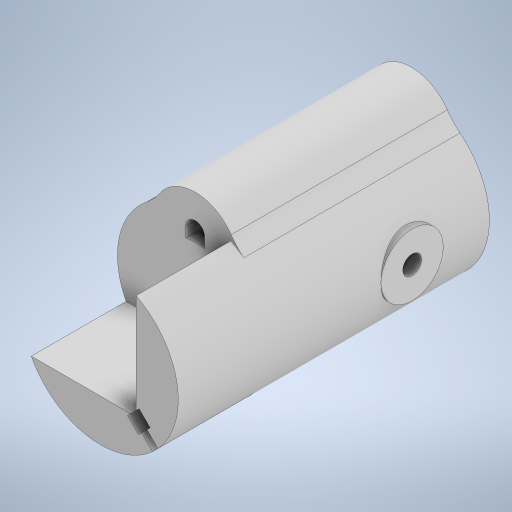
# Autodesk Inventor part: LandingFoot1
Saved by Autodesk Inventor 2023 (Build 270158000, 158)
## iProperties
Created: 2023-01-25
Part Number: LandingFoot1
Material: Generic
Document SubType Name: Modeling
Designer: chase
Density: 1 g/cm^3
Appearance: Default
Author: chase
Autodesk Inventor part; units mm, degrees
ref_plane "YZ Plane" through (0, 0, 0) normal (1, 0, 0) x (0, 1, 0)
ref_plane "XZ Plane" through (0, 0, 0) normal (0, 1, 0) x (-1, 0, 0)
ref_plane "XY Plane" through (0, 0, 0) normal (0, 0, 1) x (1, 0, 0)
sketch "Sketch1" plane through (0, 0, 0) normal (0, 0, 1) x (1, 0, 0)
  circle A0 centre (0, 0) radius 12.5
  dimension "d0" = 25
  constraints: 1 centre point
  measures "d0" diameter of A0
extrude "Extrusion1" add sketch "Sketch1" against normal blind 50
sketch "Sketch2" plane through (0, 0, 0) normal (0, 0, 1) x (1, 0, 0)
  circle A0 centre (0, 0) radius 12.5 projected
  line L0 (0, 12.5) -> (0, 0) construction
  line L1 (0, 0) -> (8.8388, -8.8388) construction
  line L2 (4.4548, -2.6163) -> (9.7581, -7.9196)
  line L3 (9.7581, -7.9196) -> (7.9196, -9.7581)
  line L4 (4.4548, -2.6163) -> (2.6163, -4.4548)
  line L5 (9.7581, -7.9196) -> (7.9196, -9.7581)
  line L6 (7.9903, -6.1518) -> (6.1518, -7.9903)
  line L7 (6.2225, -4.3841) -> (4.3841, -6.2225)
  line L8 (5.374, -4.5255) -> (4.5255, -5.374)
  line L9 (4.4194, -2.6517) -> (2.6517, -4.4194)
  line L10 (5.2679, -4.6315) -> (3.8537, -3.2173)
  line L11 (4.9497, -4.9497) -> (3.5355, -3.5355)
  line L12 (4.6315, -5.2679) -> (3.2173, -3.8537)
  line L13 (9.2631, -8.4146) -> (7.4953, -6.6468)
  line L14 (5.7276, -4.879) -> (5.374, -4.5255)
  line L15 (8.4146, -9.2631) -> (6.6468, -7.4953)
  line L16 (4.879, -5.7276) -> (4.5255, -5.374)
  line L17 (4.879, -5.7276) -> (-11.1106, -5.7276)
  line L18 (5.7276, -4.879) -> (5.7276, 11.1106)
  line L19 (3.8891, -5.7276) -> (2.6163, -4.4548)
  line L20 (7.9196, -9.7581) -> (7.8717, -9.7101)
  line L21 (6.1518, -7.9903) -> (4.3841, -6.2225)
  point P0 (7.955, -6.1872)
  point P1 (6.1872, -4.4194)
  point P2 (5.7276, -3.8891)
  point P3 (9.7101, -7.8717)
  point P4 (8.8388, -8.8388)
  dimension "d12" = 135
  dimension "d14" = 7.5
  dimension "d16" = 7.5
  dimension "d18" = 2.5
  dimension "d19" = 2.5
  dimension "d20" = 0.5
  dimension "d27" = 1.2
  dimension "d57" = 0.9
  dimension "d58" = 0.45
  dimension "d59" = 1.3
  constraints: 44 end point, 9 point on line, 6 parallel, 5 point on circle, 4 perpendicular, 2 collinear, 1 horizontal, 1 tangent, 1 vertical
  measures "d12" angle of L1 L0
  measures "d14" distance of L2.start L2.end
  measures "d16" distance of L3.end L4.end
  measures "d18" distance between parallel lines of L3 L6
  measures "d19" distance between parallel lines of L6 L7
  measures "d20" distance between parallel lines of L7 L8
  measures "d27" distance between parallel lines of L15 L13
  measures "d57" distance between parallel lines of L10 L12
  measures "d58" distance between parallel lines of L10 L1
  measures "d59" distance between parallel lines of L11 L2
sketch "Sketch3" plane through (0, 0, -50) normal (0, 0, -1) x (-1, 0, 0)
  circle A0 centre (0, 0) radius 8.075
  circle A1 centre (0, 9.575) radius 1.5
  line L0 (-1.5, 9.575) -> (-1.5, 7.9345)
  line L1 (1.5, 9.575) -> (1.5, 7.9345)
  dimension "d30" = 16.15
  dimension "d33" = 3
  constraints: 4 end point, 4 point on circle, 2 centre point, 1 coincident, 1 parallel, 1 tangent, 1 vertical
  measures "d30" diameter of A0
  measures "d33" diameter of A1
extrude "Extrusion3" cut sketch "Sketch3" against normal blind 25.4 contours A0
extrude "Extrusion4" cut sketch "Sketch3" against normal through all contours A0 A1 L1 | L0 A1 A0 | A1
sketch "Sketch4" plane through (0, 0, -50) normal (0, 0, -1) x (-1, 0, 0)
  arc A0 (6.4283, 10.7204) -> (-6.4283, 10.7204) centre (0, 8.075) ccw
  arc A1 (1.5, 7.9345) -> (-1.5, 7.9345) centre (0, 0) ccw projected
  circle A2 centre (0, 0) radius 12.5 projected
  point P0 (0, 8.075)
  dimension "d37" = 12.8567
  dimension "d38" = 6.4283
  constraints: 6 point on circle, 1 centre point
  measures "d37" distance of A0.start A0.end
  measures "d38" horizontal distance of A0.start point (0, 8.075)
ref_plane "Work Plane1" through (12.5, 0, 0) normal (-1, 0, 0) x (0, 0, 1)
sketch "Sketch6" plane through (12.5, 0, 0) normal (-1, 0, 0) x (0, 0, 1)
  circle A0 centre (-37.5833, 0) radius 5
  point P0 (0, 0)
  dimension "d48" = 10
  constraints: 1 centre point
  measures "d48" diameter of A0
ref_plane "Work Plane2" through (-12.5, 0, 0) normal (1, 0, 0) x (0, 0, -1)
extrude "Extrusion7" add sketch "Sketch6" along normal up to surface (25 mm away)
sketch "Sketch7" plane through (12.5, 0, 0) normal (1, 0, 0) x (0, 0, -1)
  arc A0 (32.5833, 0) -> (42.5833, 0) centre (37.5833, 0) ccw projected
  circle A1 centre (37.5833, 0) radius 1.5
  point P0 (0, 0)
  dimension "d51" = 3
  constraints: 1 centre point, 1 coincident
  measures "d51" diameter of A1
extrude "Extrusion8" cut sketch "Sketch7" against normal through all
sketch "Sketch8" plane through (0, 0, -50) normal (0, 0, -1) x (-1, 0, 0)
  circle A0 centre (0, 0) radius 8.075
  constraints: 1 centre point, 1 coincident
extrude "Extrusion9" cut sketch "Sketch8" against normal up to surface (25.4 mm away)
extrude "Extrusion10" cut sketch "Sketch2" against normal blind 15.24 contours L18 L2 L4 L19 L17 A0 | L18 L14 L8 L10 L4 L2 | L13 L3 A0 | A0 L15 L6 L13 | L6 L21 L7 L2 | L19 L4 L12 L8 L16 L17 | L7 L16 L8 L14 | L3 L15 A0 | L10 L8 L11 L4 | L12 L4 L11 L8
extrude "Extrusion11" add sketch "Sketch4" against normal up to surface (34.76 mm away) contours A2 A0
fillet "Fillet2" radius 10 2 edges at (6.4283, 10.7204, -32.62) (-6.4283, 10.7204, -32.62)
equation "\"d58\" = 0.5 * d57"
equation "\"d59\" = 0.5 * d56"
equation "\"d38\" = 0.5 * d37"
equation "\"d56\" = 2.6"
body "Solid1"
